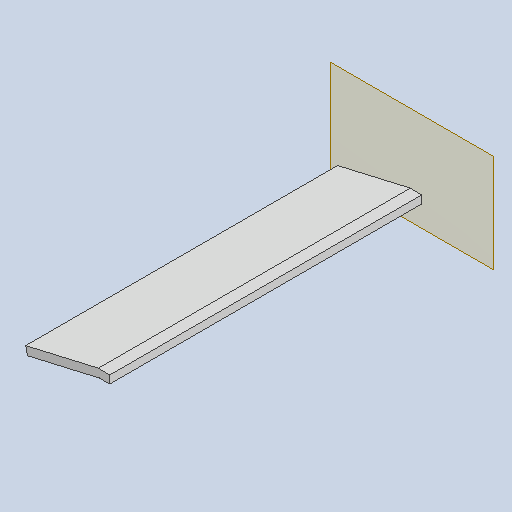
# Autodesk Inventor part: backrest
Saved by Autodesk Inventor 2023 (Build 270158030, 158C)
## iProperties
Created: 2024-09-10
Part Number: backrest
Material: Generic
Document SubType Name: Modeling
Designer: Imogen Heard
Density: 1 g/cm^3
Appearance: Default
Author: Imogen Heard
Autodesk Inventor part; units mm, degrees
ref_plane "YZ Plane" through (0, 0, 0) normal (1, 0, 0) x (0, 1, 0)
ref_plane "XZ Plane" through (0, 0, 0) normal (0, 1, 0) x (-1, 0, 0)
ref_plane "XY Plane" through (0, 0, 0) normal (0, 0, 1) x (1, 0, 0)
ref_plane "Work Plane1" through (0, 0, 0) normal (0, 0, 1) x (1, 0, 0)
sketch "Sketch1" plane through (0, 0, 0) normal (0, 0, 1) x (1, 0, 0)
  line L0 (-235, -175) -> (-685, -278.8907) projected
  line L1 (-685, -278.8907) -> (-673.7524, -327.6092) projected
  line L2 (-673.7524, -327.6092) -> (-229.3032, -225) projected
  line L3 (-165, -225) -> (-229.3032, -225) projected
  line L4 (-165, -176.5227) -> (-165, -225) projected
  line L5 (165, 54.5458) -> (-165, -176.5227) projected
  line L6 (165, -190) -> (165, 54.5458) projected
  line L7 (235, -190) -> (165, -190) projected
  line L8 (235, 190) -> (235, -190) projected
  line L9 (165, 190) -> (235, 190) projected
  line L10 (165, 140) -> (165, 190) projected
  line L11 (-165, -91.0685) -> (165, 140) projected
  line L12 (-165, 225) -> (-165, -91.0685) projected
  line L13 (-235, 225) -> (-165, 225) projected
  line L14 (-235, -175) -> (-235, 225) projected
  arc A0 (-195, -120) -> (-205, -110) centre (-205, -120) ccw projected
  line L15 (-195, -120) -> (-195, -160) projected
  arc A1 (-205, -170) -> (-195, -160) centre (-205, -160) ccw projected
  line L16 (-205, -170) -> (-215, -170) projected
  arc A2 (-225, -160) -> (-215, -170) centre (-215, -160) ccw projected
  line L17 (-225, -160) -> (-225, -120) projected
  arc A3 (-215, -110) -> (-225, -120) centre (-215, -120) ccw projected
  line L18 (-215, -110) -> (-205, -110) projected
  arc A4 (-195, 140) -> (-205, 150) centre (-205, 140) ccw projected
  line L19 (-195, 140) -> (-195, 100) projected
  arc A5 (-205, 90) -> (-195, 100) centre (-205, 100) ccw projected
  line L20 (-205, 90) -> (-215, 90) projected
  arc A6 (-225, 100) -> (-215, 90) centre (-215, 100) ccw projected
  line L21 (-225, 100) -> (-225, 140) projected
  arc A7 (-215, 150) -> (-225, 140) centre (-215, 140) ccw projected
  line L22 (-215, 150) -> (-205, 150) projected
  arc A8 (-195, 75) -> (-205, 85) centre (-205, 75) ccw projected
  line L23 (-195, 75) -> (-195, 35) projected
  arc A9 (-205, 25) -> (-195, 35) centre (-205, 35) ccw projected
  line L24 (-205, 25) -> (-215, 25) projected
  arc A10 (-225, 35) -> (-215, 25) centre (-215, 35) ccw projected
  line L25 (-225, 35) -> (-225, 75) projected
  arc A11 (-215, 85) -> (-225, 75) centre (-215, 75) ccw projected
  line L26 (-215, 85) -> (-205, 85) projected
  arc A12 (-195, -55) -> (-205, -45) centre (-205, -55) ccw projected
  line L27 (-195, -55) -> (-195, -95) projected
  arc A13 (-205, -105) -> (-195, -95) centre (-205, -95) ccw projected
  line L28 (-205, -105) -> (-215, -105) projected
  arc A14 (-225, -95) -> (-215, -105) centre (-215, -95) ccw projected
  line L29 (-225, -95) -> (-225, -55) projected
  arc A15 (-215, -45) -> (-225, -55) centre (-215, -55) ccw projected
  line L30 (-215, -45) -> (-205, -45) projected
  arc A16 (-195, 205) -> (-205, 215) centre (-205, 205) ccw projected
  line L31 (-195, 205) -> (-195, 165) projected
  arc A17 (-205, 155) -> (-195, 165) centre (-205, 165) ccw projected
  line L32 (-205, 155) -> (-215, 155) projected
  arc A18 (-225, 165) -> (-215, 155) centre (-215, 165) ccw projected
  line L33 (-225, 165) -> (-225, 205) projected
  arc A19 (-215, 215) -> (-225, 205) centre (-215, 205) ccw projected
  line L34 (-215, 215) -> (-205, 215) projected
  arc A20 (-195, 10) -> (-205, 20) centre (-205, 10) ccw projected
  line L35 (-195, 10) -> (-195, -30) projected
  arc A21 (-205, -40) -> (-195, -30) centre (-205, -30) ccw projected
  line L36 (-205, -40) -> (-215, -40) projected
  arc A22 (-225, -30) -> (-215, -40) centre (-215, -30) ccw projected
  line L37 (-225, -30) -> (-225, 10) projected
  arc A23 (-215, 20) -> (-225, 10) centre (-215, 10) ccw projected
  line L38 (-215, 20) -> (-205, 20) projected
  line L39 (-235, -175) -> (-165, -176.5227)
  point P0 (0, 0)
  constraints: 2 end point, 1 other
extrude "Extrusion1" add sketch "Sketch1" along normal blind 1930 contours L39 L4 L3 L2 L1 L0
